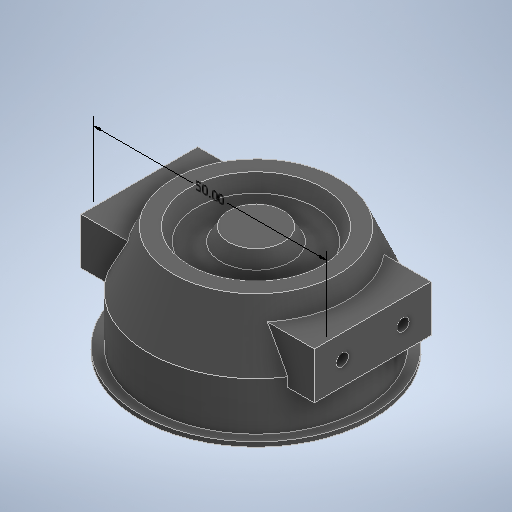
# Autodesk Inventor part: volume_handle
Saved by Autodesk Inventor 2026.1 (Build 301233020, 233B)
## iProperties
Created: 2026-02-01
Part Number: volume_handle
Material: 一般
Document SubType Name: Modeling
Designer: hibik
Density: 1 g/cm^3
Appearance: 既定
Author: hibik
Autodesk Inventor part; units mm, degrees
ref_plane "XZ Plane" through (0, 0, 0) normal (0, 1, 0) x (-1, 0, 0)
ref_plane "XY Plane" through (0, 0, 0) normal (0, 0, 1) x (1, 0, 0)
sketch "スケッチ1" plane through (0, 0, 0) normal (0, 1, 0) x (-1, 0, 0)
  circle A0 centre (0, 0) radius 23
  dimension "d0" = 46
  constraints: 1 centre point, 1 coincident
  measures "d0" diameter of A0
extrude "押し出し1" add sketch "スケッチ1" along normal blind 24
shell "シェル1" thickness 1.5 removed faces 1 at (-0.3013, 0, 5.0839)
sketch "スケッチ2" plane through (0, 22.5, 0) normal (0, -1, 0) x (1, 0, 0)
  circle A0 centre (0, 0) radius 5
  dimension "d5" = 10
  constraints: 1 centre point, 1 coincident
  measures "d5" diameter of A0
extrude "押し出し2" add sketch "スケッチ2" along normal blind 13
sketch "スケッチ3" plane through (0, 22.5, 0) normal (0, -1, 0) x (1, 0, 0)
  circle A0 centre (0, 0) radius 3
  dimension "d8" = 6
  constraints: 1 centre point, 1 coincident
  measures "d8" diameter of A0
extrude "押し出し3" cut sketch "スケッチ3" along normal through all draft 1.2
sketch "スケッチ4" plane through (0, 9.5, 0) normal (0, -1, 0) x (1, 0, 0)
  circle A0 centre (0, -3.2723) radius 0.25
  circle A1 centre (0, 0) radius 3.2723 construction
  dimension "d13" = 0.5
  constraints: 2 vertical alignment, 1 centre point, 1 other
  measures "d13" diameter of A0
extrude "押し出し4" add sketch "スケッチ4" against normal up to surface (13 mm away) draft 0.3
pattern_circular "円形状パターン1" count 18 over 360 about axis through (0, -10, 0) along (0, 1, 0) of "押し出し4"
sketch "スケッチ6" plane through (0, 0, 0) normal (1, 0, 0) x (0, 1, 0)
  line L0 (24, -23) -> (0, -23) projected
  line L1 (0, -23) -> (0, -21.5) projected
  line L2 (0, -21.5) -> (22.5, -21.5) projected
  line L3 (22.5, -21.5) -> (22.5, -5) projected
  line L4 (22.5, -5) -> (9.5, -5) projected
  line L5 (9.5, -5) -> (9.5, -3.0223) projected
  line L6 (9.5, -3.0223) -> (22.5, -2.9542) projected
  line L7 (22.5, -2.9542) -> (22.5, 2.9542) projected
  line L8 (22.5, 2.9542) -> (9.5, 3.0223) projected
  line L9 (9.5, 3.0223) -> (9.5, 5) projected
  line L10 (9.5, 5) -> (22.5, 5) projected
  line L11 (22.5, 5) -> (22.5, 21.5) projected
  line L12 (22.5, 21.5) -> (0, 21.5) projected
  line L13 (0, 21.5) -> (0, 23) projected
  line L14 (0, 23) -> (24, 23) projected
  line L15 (24, 23) -> (24, -23) projected
  line L16 (24, 5.866) -> (19.5, 8.4641)
  line L17 (19.5, 8.4641) -> (19.5, 11.7321)
  line L18 (19.5, 11.7321) -> (24, 14.3301)
  line L19 (24, 4.134) -> (18, 7.5981)
  line L20 (18, 7.5981) -> (18, 12.5981)
  line L21 (18, 12.5981) -> (24, 16.0622)
  line L22 (24, 17.7019) -> (12, 23)
  line L23 (22.5, 16.7244) -> (11.6836, 21.5)
  line L24 (19.5, 10.0981) -> (18, 10.0981)
  line L25 (-4.2, 0) -> (25.2, 0) projected
  point P0 (0, 0)
  point P1 (22.5, 18.3641)
  point P2 (15.3974, 21.5)
  point P3 (22.5, 6.7321)
  point P4 (22.5, 13.4641)
  point P5 (22.5, 15.1962)
  point P6 (0, 22.25)
  dimension "d19" = 1.5
  dimension "d20" = 1.5
  dimension "d21" = 1.5
  dimension "d22" = 1.5
  dimension "d23" = 60
  dimension "d24" = 5
  dimension "d25" = 3
  dimension "d35" = 12
  constraints: 18 end point, 9 point on line, 4 midpoint, 4 parallel, 1 perpendicular, 1 vertical
  measures "d19" distance between parallel lines of L16 L19
  measures "d20" distance between parallel lines of L20 L17
  measures "d21" distance between parallel lines of L21 L18
  measures "d22" distance between parallel lines of L22 L23
  measures "d23" angle of L11 L16
  measures "d24" distance of L19.end L20.end
  measures "d25" distance between parallel lines of L11 L17
  measures "d35" horizontal distance of point (0, 22.25) L22.end
revolve "回転1" cut sketch "スケッチ6" angle 360 about axis through (0, -10, 0) along (0, 1, 0) contours L16 L11 L18 L15 | L16 L17 L18 L11 | L22 L11 L12 L14 L15 | L22 L12 L11
revolve "回転2" add sketch "スケッチ6" angle 360 about axis through (0, -10, 0) along (0, 1, 0) contours L19 L20 L24 L17 L16 L11 | L18 L17 L24 L20 L21 L11 | L11 L23 L12 L22
fillet "フィレット1" radius 2 2 edges at (3.5355, 22.5, 3.5355) (-3.5355, 22.5, -3.5355)
ref_plane "作業平面2" through (25, 0, 0) normal (1, 0, 0) x (0, 1, 0)
ref_plane "作業平面1" through (23, 0, 0) normal (1, 0, 0) x (0, 1, 0)
sketch "スケッチ7" plane through (25, 0, 0) normal (1, 0, 0) x (0, 1, 0)
  line L0 (20, 12.5) -> (10, 12.5)
  line L1 (10, 12.5) -> (10, -12.5)
  line L2 (10, -12.5) -> (20, -12.5)
  line L3 (20, -12.5) -> (20, 12.5)
  line L4 (24, -17.7019) -> (24, 17.7019) projected
  line L5 (12, 23) -> (12, -23) projected
  point P0 (10, 0)
  point P1 (10, 0)
  point P2 (0, 0)
  point P3 (12, 12.5)
  point P4 (12, -12.5)
  dimension "d31" = 25
  dimension "d41" = 4
  dimension "d42" = 10
  constraints: 8 end point, 2 midpoint, 2 parallel, 1 coincident, 1 horizontal, 1 horizontal alignment, 1 perpendicular
  measures "d31" distance of L2.end L0.start
  measures "d41" distance between parallel lines of L4 L3
  measures "d42" distance of L0.start L0.end
extrude "押し出し5" add sketch "スケッチ7" against normal up to surface round surface about axis through (0, 0, 0) along (0, 1, 0) radius 23 far side no
sketch "スケッチ8" plane through (25, 0, 0) normal (1, 0, 0) x (0, 0, -1)
  circle A0 centre (-6.5, 15) radius 1.3
  circle A1 centre (6.5, 15) radius 1.3
  line L0 (12.5, 20) -> (-12.5, 20) construction
  line L1 (-12.5, 20) -> (-12.5, 10) construction
  line L2 (0, 20) -> (0, 0) construction
  point P0 (-12.5, 15)
  dimension "d36" = 2.6
  dimension "d38" = 6
  constraints: 2 centre point, 2 end point, 2 horizontal alignment, 2 midpoint, 1 vertical, 1 other
  measures "d36" diameter of A0
  measures "d38" distance from line of L1 A0.centre
extrude "押し出し7" add sketch "スケッチ7" against normal up to surface contours L3 L2 L5 L0 round surface about axis through (0, 18, 0) along (0, -1, 0) radius 20.3509 half angle 23.821971 far side no
extrude "押し出し8" cut sketch "スケッチ8" against normal blind 13
mirror "ミラー2" about plane through (0, 0, 0) normal (1, 0, 0) of "押し出し5", "押し出し7", "押し出し8"
fillet "フィレット2" radius 3 2 edges at (0, 19.5, -8.4641) (0, 19.5, -11.7321)
ref_plane "作業平面3" through (0, 0.7, 0) normal (0, -1, 0) x (1, 0, 0)
sketch "スケッチ9" plane through (0, 0.7, 0) normal (0, -1, 0) x (1, 0, 0)
  circle A0 centre (0, 0) radius 23 projected
  circle A1 centre (0, 0) radius 25
  dimension "d52" = 2
  constraints: 1 centre point, 1 coincident
  measures "d52" radial gap between concentric circles of A1 A0
extrude "押し出し9" add sketch "スケッチ9" against normal blind 1
equation "\"d20\" = d19"
equation "\"d21\" = d19"
equation "\"d22\" = d21"
